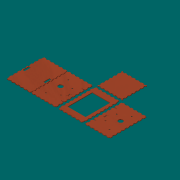
# Autodesk Inventor part: panelsWithKerf
Saved by Autodesk Inventor 2016 SP2 (Build 200236200, 236)
## iProperties
Created: 2016-09-07
Part Number: panelsWithKerf
Material: Generic
Document SubType Name: Modeling
Designer: sawaiz
Density: 1 g/cm^3
Appearance: Copper - Satin
Author: sawaiz
Autodesk Inventor part; units mm, degrees
(part 1 of 2)
ref_plane "YZ Plane" through (0, 0, 0) normal (1, 0, 0) x (0, 1, 0)
ref_plane "XZ Plane" through (0, 0, 0) normal (0, 1, 0) x (-1, 0, 0)
ref_plane "XY Plane" through (0, 0, 0) normal (0, 0, 1) x (1, 0, 0)
sketch "Sketch2" plane through (0, 0, 0) normal (0, 0, 1) x (1, 0, 0)
  line L0 (-285.4, 15) -> (-285.4, -15) construction
  line L1 (-285.4, -15) -> (-295.4, -15) construction
  line L2 (-295.4, -15) -> (-295.4, 15) construction
  line L3 (-295.4, 15) -> (-285.4, 15) construction
  line L4 (-185.4, 15) -> (-185.4, -15) construction
  line L5 (-185.4, -15) -> (-195.4, -15) construction
  line L6 (-195.4, -15) -> (-195.4, 15) construction
  line L7 (-195.4, 15) -> (-185.4, 15) construction
  circle A0 centre (-297.225, -50) radius 1.7 projected
  circle A1 centre (-297.225, 50) radius 1.7 projected
  circle A2 centre (-183.575, -50) radius 1.7 projected
  circle A3 centre (-183.575, 50) radius 1.7 projected
  line L8 (-297.225, 86.825) -> (-297.225, 75) construction
  line L9 (-297.225, 75) -> (-300.4, 75) construction
  line L10 (-300.4, 75) -> (-300.4, 65) construction
  line L11 (-300.4, 65) -> (-297.225, 65) construction
  line L12 (-297.225, 65) -> (-297.225, 55) construction
  line L13 (-297.225, 55) -> (-300.4, 55) construction
  line L14 (-300.4, 55) -> (-300.4, 45) construction
  line L15 (-300.4, 45) -> (-297.225, 45) construction
  line L16 (-297.225, 45) -> (-297.225, 35) construction
  line L17 (-297.225, 35) -> (-300.4, 35) construction
  line L18 (-300.4, 35) -> (-300.4, 25) construction
  line L19 (-300.4, 25) -> (-297.225, 25) construction
  line L20 (-297.225, 25) -> (-297.225, 15) construction
  line L21 (-297.225, 15) -> (-300.4, 15) construction
  line L22 (-300.4, 15) -> (-300.4, 5) construction
  line L23 (-300.4, 5) -> (-297.225, 5) construction
  line L24 (-297.225, 5) -> (-297.225, -5) construction
  line L25 (-297.225, -5) -> (-300.4, -5) construction
  line L26 (-300.4, -5) -> (-300.4, -15) construction
  line L27 (-300.4, -15) -> (-297.225, -15) construction
  line L28 (-297.225, -15) -> (-297.225, -25) construction
  line L29 (-297.225, -25) -> (-300.4, -25) construction
  line L30 (-300.4, -25) -> (-300.4, -35) construction
  line L31 (-300.4, -35) -> (-297.225, -35) construction
  line L32 (-297.225, -35) -> (-297.225, -45) construction
  line L33 (-297.225, -45) -> (-300.4, -45) construction
  line L34 (-300.4, -45) -> (-300.4, -55) construction
  line L35 (-300.4, -55) -> (-297.225, -55) construction
  line L36 (-297.225, -55) -> (-297.225, -65) construction
  line L37 (-297.225, -65) -> (-300.4, -65) construction
  line L38 (-300.4, -65) -> (-300.4, -75) construction
  line L39 (-300.4, -75) -> (-297.225, -75) construction
  line L40 (-297.225, -75) -> (-297.225, -86.825) construction
  line L41 (-297.225, -86.825) -> (-295.4, -86.825) construction
  line L42 (-295.4, -86.825) -> (-295.4, -90) construction
  line L43 (-295.4, -90) -> (-285.4, -90) construction
  line L44 (-285.4, -90) -> (-285.4, -86.825) construction
  line L45 (-285.4, -86.825) -> (-275.4, -86.825) construction
  line L46 (-275.4, -86.825) -> (-275.4, -90) construction
  line L47 (-275.4, -90) -> (-265.4, -90) construction
  line L48 (-265.4, -90) -> (-265.4, -86.825) construction
  line L49 (-265.4, -86.825) -> (-255.4, -86.825) construction
  line L50 (-255.4, -86.825) -> (-255.4, -90) construction
  line L51 (-255.4, -90) -> (-245.4, -90) construction
  line L52 (-245.4, -90) -> (-245.4, -86.825) construction
  line L53 (-245.4, -86.825) -> (-235.4, -86.825) construction
  line L54 (-235.4, -86.825) -> (-235.4, -90) construction
  line L55 (-235.4, -90) -> (-225.4, -90) construction
  line L56 (-225.4, -90) -> (-225.4, -86.825) construction
  line L57 (-225.4, -86.825) -> (-215.4, -86.825) construction
  line L58 (-215.4, -86.825) -> (-215.4, -90) construction
  line L59 (-215.4, -90) -> (-205.4, -90) construction
  line L60 (-205.4, -90) -> (-205.4, -86.825) construction
  line L61 (-205.4, -86.825) -> (-195.4, -86.825) construction
  line L62 (-195.4, -86.825) -> (-195.4, -90) construction
  line L63 (-195.4, -90) -> (-185.4, -90) construction
  line L64 (-185.4, -90) -> (-185.4, -86.825) construction
  line L65 (-185.4, -86.825) -> (-183.575, -86.825) construction
  line L66 (-183.575, -86.825) -> (-183.575, -75) construction
  line L67 (-183.575, -75) -> (-180.4, -75) construction
  line L68 (-180.4, -75) -> (-180.4, -65) construction
  line L69 (-180.4, -65) -> (-183.575, -65) construction
  line L70 (-183.575, -65) -> (-183.575, -55) construction
  line L71 (-183.575, -55) -> (-180.4, -55) construction
  line L72 (-180.4, -55) -> (-180.4, -45) construction
  line L73 (-180.4, -45) -> (-183.575, -45) construction
  line L74 (-183.575, -45) -> (-183.575, -35) construction
  line L75 (-183.575, -35) -> (-180.4, -35) construction
  line L76 (-180.4, -35) -> (-180.4, -25) construction
  line L77 (-180.4, -25) -> (-183.575, -25) construction
  line L78 (-183.575, -25) -> (-183.575, -15) construction
  line L79 (-183.575, -15) -> (-180.4, -15) construction
  line L80 (-180.4, -15) -> (-180.4, -5) construction
  line L81 (-180.4, -5) -> (-183.575, -5) construction
  line L82 (-183.575, -5) -> (-183.575, 5) construction
  line L83 (-183.575, 5) -> (-180.4, 5) construction
  line L84 (-180.4, 5) -> (-180.4, 15) construction
  line L85 (-180.4, 15) -> (-183.575, 15) construction
  line L86 (-183.575, 15) -> (-183.575, 25) construction
  line L87 (-183.575, 25) -> (-180.4, 25) construction
  line L88 (-180.4, 25) -> (-180.4, 35) construction
  line L89 (-180.4, 35) -> (-183.575, 35) construction
  line L90 (-183.575, 35) -> (-183.575, 45) construction
  line L91 (-183.575, 45) -> (-180.4, 45) construction
  line L92 (-180.4, 45) -> (-180.4, 55) construction
  line L93 (-180.4, 55) -> (-183.575, 55) construction
  line L94 (-183.575, 55) -> (-183.575, 65) construction
  line L95 (-183.575, 65) -> (-180.4, 65) construction
  line L96 (-180.4, 65) -> (-180.4, 75) construction
  line L97 (-180.4, 75) -> (-183.575, 75) construction
  line L98 (-183.575, 75) -> (-183.575, 86.825) construction
  line L99 (-183.575, 86.825) -> (-185.4, 86.825) construction
  line L100 (-185.4, 86.825) -> (-185.4, 90) construction
  line L101 (-185.4, 90) -> (-195.4, 90) construction
  line L102 (-195.4, 90) -> (-195.4, 86.825) construction
  line L103 (-195.4, 86.825) -> (-205.4, 86.825) construction
  line L104 (-205.4, 86.825) -> (-205.4, 90) construction
  line L105 (-205.4, 90) -> (-215.4, 90) construction
  line L106 (-215.4, 90) -> (-215.4, 86.825) construction
  line L107 (-215.4, 86.825) -> (-225.4, 86.825) construction
  line L108 (-225.4, 86.825) -> (-225.4, 90) construction
  line L109 (-225.4, 90) -> (-235.4, 90) construction
  line L110 (-235.4, 90) -> (-235.4, 86.825) construction
  line L111 (-235.4, 86.825) -> (-245.4, 86.825) construction
  line L112 (-245.4, 86.825) -> (-245.4, 90) construction
  line L113 (-245.4, 90) -> (-255.4, 90) construction
  line L114 (-255.4, 90) -> (-255.4, 86.825) construction
  line L115 (-255.4, 86.825) -> (-265.4, 86.825) construction
  line L116 (-265.4, 86.825) -> (-265.4, 90) construction
  line L117 (-265.4, 90) -> (-275.4, 90) construction
  line L118 (-275.4, 90) -> (-275.4, 86.825) construction
  line L119 (-275.4, 86.825) -> (-285.4, 86.825) construction
  line L120 (-285.4, 86.825) -> (-285.4, 90) construction
  line L121 (-285.4, 90) -> (-295.4, 90) construction
  line L122 (-295.4, 90) -> (-295.4, 86.825) construction
  line L123 (-295.4, 86.825) -> (-297.225, 86.825) construction
  line L124 (-76.385, -13.335) -> (-80.195, -13.335) projected
  line L125 (-80.195, -13.335) -> (-80.195, -1.905) projected
  line L126 (-80.195, -1.905) -> (-76.385, -1.905) projected
  line L127 (-76.385, -1.905) -> (-76.385, -13.335) projected
  circle A4 centre (-82.1, -15.24) radius 1.078 projected
  circle A5 centre (-74.48, 0) radius 1.078 projected
  circle A6 centre (-74.48, -15.24) radius 1.078 projected
  circle A7 centre (-82.1, 0) radius 1.078 projected
  line L128 (-65.375, -48.5) -> (-63.375, -48.5) construction
  line L129 (-63.375, -48.5) -> (-63.375, -45) construction
  line L130 (-63.375, -45) -> (-60.2, -45) construction
  line L131 (-60.2, -45) -> (-60.2, -35) construction
  line L132 (-60.2, -35) -> (-63.375, -35) construction
  line L133 (-63.375, -35) -> (-63.375, -25) construction
  line L134 (-63.375, -25) -> (-60.2, -25) construction
  line L135 (-60.2, -25) -> (-60.2, -15) construction
  line L136 (-60.2, -15) -> (-63.375, -15) construction
  line L137 (-63.375, -15) -> (-63.375, -5) construction
  line L138 (-63.375, -5) -> (-60.2, -5) construction
  line L139 (-60.2, -5) -> (-60.2, 5) construction
  line L140 (-60.2, 5) -> (-63.375, 5) construction
  line L141 (-63.375, 5) -> (-63.375, 15) construction
  line L142 (-63.375, 15) -> (-60.2, 15) construction
  line L143 (-60.2, 15) -> (-60.2, 25) construction
  line L144 (-60.2, 25) -> (-63.375, 25) construction
  line L145 (-63.375, 25) -> (-63.375, 35) construction
  line L146 (-63.375, 35) -> (-60.2, 35) construction
  line L147 (-60.2, 35) -> (-60.2, 45) construction
  line L148 (-60.2, 45) -> (-63.375, 45) construction
  line L149 (-63.375, 45) -> (-63.375, 48.5) construction
  line L150 (-63.375, 48.5) -> (-65.375, 48.5) construction
  line L151 (-65.375, 48.5) -> (-65.375, 47.25) construction
  line L152 (-65.375, 47.25) -> (-67.875, 47.25) construction
  line L153 (-67.875, 47.25) -> (-67.875, 48.5) construction
  line L154 (-67.875, 48.5) -> (-74.2, 48.5) construction
  line L155 (-74.2, 48.5) -> (-74.2, 51.5) construction
  line L156 (-74.2, 51.5) -> (-67.875, 51.5) construction
  line L157 (-67.875, 51.5) -> (-67.875, 52.75) construction
  line L158 (-67.875, 52.75) -> (-65.375, 52.75) construction
  line L159 (-65.375, 52.75) -> (-65.375, 51.5) construction
  line L160 (-65.375, 51.5) -> (-63.375, 51.5) construction
  line L161 (-63.375, 51.5) -> (-63.375, 55) construction
  line L162 (-63.375, 55) -> (-60.2, 55) construction
  line L163 (-60.2, 55) -> (-60.2, 65) construction
  line L164 (-60.2, 65) -> (-63.375, 65) construction
  line L165 (-63.375, 65) -> (-63.375, 75) construction
  line L166 (-63.375, 75) -> (-60.2, 75) construction
  line L167 (-60.2, 75) -> (-60.2, 86.825) construction
  line L168 (-65.2, 86.825) -> (-60.2, 86.825) construction
  line L169 (-65.2, 90) -> (-65.2, 86.825) construction
  line L170 (-75.2, 90) -> (-65.2, 90) construction
  line L171 (-75.2, 86.825) -> (-75.2, 90) construction
  line L172 (-75.2, 86.825) -> (-85.2, 86.825) construction
  line L173 (-85.2, 90) -> (-85.2, 86.825) construction
  line L174 (-95.2, 90) -> (-85.2, 90) construction
  line L175 (-95.2, 86.825) -> (-95.2, 90) construction
  line L176 (-95.2, 86.825) -> (-105.2, 86.825) construction
  line L177 (-105.2, 90) -> (-105.2, 86.825) construction
  line L178 (-115.2, 90) -> (-105.2, 90) construction
  line L179 (-115.2, 86.825) -> (-115.2, 90) construction
  line L180 (-115.2, 86.825) -> (-125.2, 86.825) construction
  line L181 (-125.2, 90) -> (-125.2, 86.825) construction
  line L182 (-135.2, 90) -> (-125.2, 90) construction
  line L183 (-135.2, 86.825) -> (-135.2, 90) construction
  line L184 (-135.2, 86.825) -> (-145.2, 86.825) construction
  line L185 (-145.2, 90) -> (-145.2, 86.825) construction
  line L186 (-155.2, 90) -> (-145.2, 90) construction
  line L187 (-155.2, 86.825) -> (-155.2, 90) construction
  line L188 (-155.2, 86.825) -> (-165.2, 86.825) construction
  line L189 (-165.2, 90) -> (-165.2, 86.825) construction
  line L190 (-175.2, 90) -> (-165.2, 90) construction
  line L191 (-175.2, 86.825) -> (-175.2, 90) construction
  line L192 (-175.2, 86.825) -> (-180.2, 86.825) construction
  line L193 (-180.2, 75) -> (-180.2, 86.825) construction
  line L194 (-177.025, 75) -> (-180.2, 75) construction
  line L195 (-177.025, 75) -> (-177.025, 65) construction
  line L196 (-180.2, 65) -> (-177.025, 65) construction
  line L197 (-180.2, 55) -> (-180.2, 65) construction
  line L198 (-177.025, 55) -> (-180.2, 55) construction
  line L199 (-177.025, 55) -> (-177.025, 45) construction
  line L200 (-180.2, 45) -> (-177.025, 45) construction
  line L201 (-180.2, 35) -> (-180.2, 45) construction
  line L202 (-177.025, 35) -> (-180.2, 35) construction
  line L203 (-177.025, 35) -> (-177.025, 25) construction
  line L204 (-180.2, 25) -> (-177.025, 25) construction
  line L205 (-180.2, 15) -> (-180.2, 25) construction
  line L206 (-177.025, 15) -> (-180.2, 15) construction
  line L207 (-177.025, 15) -> (-177.025, 5) construction
  line L208 (-180.2, 5) -> (-177.025, 5) construction
  line L209 (-180.2, -5) -> (-180.2, 5) construction
  line L210 (-177.025, -5) -> (-180.2, -5) construction
  line L211 (-177.025, -5) -> (-177.025, -15) construction
  line L212 (-180.2, -15) -> (-177.025, -15) construction
  line L213 (-180.2, -25) -> (-180.2, -15) construction
  line L214 (-177.025, -25) -> (-180.2, -25) construction
  line L215 (-177.025, -25) -> (-177.025, -35) construction
  line L216 (-180.2, -35) -> (-177.025, -35) construction
  line L217 (-180.2, -45) -> (-180.2, -35) construction
  line L218 (-177.025, -45) -> (-180.2, -45) construction
  line L219 (-177.025, -45) -> (-177.025, -55) construction
  line L220 (-180.2, -55) -> (-177.025, -55) construction
  line L221 (-180.2, -65) -> (-180.2, -55) construction
  line L222 (-177.025, -65) -> (-180.2, -65) construction
  line L223 (-177.025, -65) -> (-177.025, -75) construction
  line L224 (-180.2, -75) -> (-177.025, -75) construction
  line L225 (-180.2, -75) -> (-180.2, -86.825) construction
  line L226 (-180.2, -86.825) -> (-175.2, -86.825) construction
  line L227 (-175.2, -86.825) -> (-175.2, -90) construction
  line L228 (-175.2, -90) -> (-165.2, -90) construction
  line L229 (-165.2, -90) -> (-165.2, -86.825) construction
  line L230 (-165.2, -86.825) -> (-155.2, -86.825) construction
  line L231 (-155.2, -86.825) -> (-155.2, -90) construction
  line L232 (-155.2, -90) -> (-145.2, -90) construction
  line L233 (-145.2, -90) -> (-145.2, -86.825) construction
  line L234 (-145.2, -86.825) -> (-135.2, -86.825) construction
  line L235 (-135.2, -86.825) -> (-135.2, -90) construction
  line L236 (-135.2, -90) -> (-125.2, -90) construction
  line L237 (-125.2, -90) -> (-125.2, -86.825) construction
  line L238 (-125.2, -86.825) -> (-115.2, -86.825) construction
  line L239 (-115.2, -86.825) -> (-115.2, -90) construction
  line L240 (-115.2, -90) -> (-105.2, -90) construction
  line L241 (-105.2, -90) -> (-105.2, -86.825) construction
  line L242 (-105.2, -86.825) -> (-95.2, -86.825) construction
  line L243 (-95.2, -86.825) -> (-95.2, -90) construction
  line L244 (-95.2, -90) -> (-85.2, -90) construction
  line L245 (-85.2, -90) -> (-85.2, -86.825) construction
  line L246 (-85.2, -86.825) -> (-75.2, -86.825) construction
  line L247 (-75.2, -86.825) -> (-75.2, -90) construction
  line L248 (-75.2, -90) -> (-65.2, -90) construction
  line L249 (-65.2, -90) -> (-65.2, -86.825) construction
  line L250 (-65.2, -86.825) -> (-60.2, -86.825) construction
  line L251 (-60.2, -86.825) -> (-60.2, -75) construction
  line L252 (-60.2, -75) -> (-63.375, -75) construction
  line L253 (-63.375, -75) -> (-63.375, -65) construction
  line L254 (-63.375, -65) -> (-60.2, -65) construction
  line L255 (-60.2, -65) -> (-60.2, -55) construction
  line L256 (-60.2, -55) -> (-63.375, -55) construction
  line L257 (-63.375, -55) -> (-63.375, -51.5) construction
  line L258 (-63.375, -51.5) -> (-65.375, -51.5) construction
  line L259 (-65.375, -51.5) -> (-65.375, -52.75) construction
  line L260 (-65.375, -52.75) -> (-67.875, -52.75) construction
  line L261 (-67.875, -52.75) -> (-67.875, -51.5) construction
  line L262 (-67.875, -51.5) -> (-74.2, -51.5) construction
  line L263 (-74.2, -51.5) -> (-74.2, -48.5) construction
  line L264 (-74.2, -48.5) -> (-67.875, -48.5) construction
  line L265 (-67.875, -48.5) -> (-67.875, -47.25) construction
  line L266 (-67.875, -47.25) -> (-65.375, -47.25) construction
  line L267 (-65.375, -47.25) -> (-65.375, -48.5) construction
  circle A8 centre (-97.2028, -27.4451) radius 3 projected
  circle A9 centre (-143.1972, 54) radius 3 projected
  circle A10 centre (-97.2028, 27.4451) radius 3 projected
  circle A11 centre (-143.1972, -54) radius 3 projected
  circle A12 centre (-135.2, 8.175) radius 11 projected
  line L268 (43.8, 60) -> (43.8, -60) construction
  line L269 (43.8, -60) -> (-43.8, -60) construction
  line L270 (-43.8, -60) -> (-43.8, 60) construction
  line L271 (-43.8, 60) -> (43.8, 60) construction
  line L272 (-56.825, 86.825) -> (-56.825, 75) construction
  line L273 (-56.825, 75) -> (-60, 75) construction
  line L274 (-60, 75) -> (-60, 65) construction
  line L275 (-60, 65) -> (-56.825, 65) construction
  line L276 (-56.825, 65) -> (-56.825, 55) construction
  line L277 (-56.825, 55) -> (-60, 55) construction
  line L278 (-60, 55) -> (-60, 45) construction
  line L279 (-60, 45) -> (-56.825, 45) construction
  line L280 (-56.825, 45) -> (-56.825, 35) construction
  line L281 (-56.825, 35) -> (-60, 35) construction
  line L282 (-60, 35) -> (-60, 25) construction
  line L283 (-60, 25) -> (-56.825, 25) construction
  line L284 (-56.825, 25) -> (-56.825, 15) construction
  line L285 (-56.825, 15) -> (-60, 15) construction
  line L286 (-60, 15) -> (-60, 5) construction
  line L287 (-60, 5) -> (-56.825, 5) construction
  line L288 (-56.825, 5) -> (-56.825, -5) construction
  line L289 (-56.825, -5) -> (-60, -5) construction
  line L290 (-60, -5) -> (-60, -15) construction
  line L291 (-60, -15) -> (-56.825, -15) construction
  line L292 (-56.825, -15) -> (-56.825, -25) construction
  line L293 (-56.825, -25) -> (-60, -25) construction
  line L294 (-60, -25) -> (-60, -35) construction
  line L295 (-60, -35) -> (-56.825, -35) construction
  line L296 (-56.825, -35) -> (-56.825, -45) construction
  line L297 (-56.825, -45) -> (-60, -45) construction
  line L298 (-60, -45) -> (-60, -55) construction
  line L299 (-60, -55) -> (-56.825, -55) construction
  line L300 (-56.825, -55) -> (-56.825, -65) construction
  line L301 (-56.825, -65) -> (-60, -65) construction
  line L302 (-60, -65) -> (-60, -75) construction
  line L303 (-60, -75) -> (-56.825, -75) construction
  line L304 (-56.825, -75) -> (-56.825, -86.825) construction
  line L305 (-56.825, -86.825) -> (-55, -86.825) construction
  line L306 (-55, -86.825) -> (-55, -90) construction
  line L307 (-55, -90) -> (-45, -90) construction
  line L308 (-45, -90) -> (-45, -86.825) construction
  line L309 (-45, -86.825) -> (-35, -86.825) construction
  line L310 (-35, -86.825) -> (-35, -90) construction
  line L311 (-35, -90) -> (-25, -90) construction
  line L312 (-25, -90) -> (-25, -86.825) construction
  line L313 (-25, -86.825) -> (-15, -86.825) construction
  line L314 (-15, -86.825) -> (-15, -90) construction
  line L315 (-15, -90) -> (-5, -90) construction
  line L316 (-5, -90) -> (-5, -86.825) construction
  line L317 (-5, -86.825) -> (5, -86.825) construction
  line L318 (5, -86.825) -> (5, -90) construction
  line L319 (5, -90) -> (15, -90) construction
  line L320 (15, -90) -> (15, -86.825) construction
  line L321 (15, -86.825) -> (25, -86.825) construction
  line L322 (25, -86.825) -> (25, -90) construction
  line L323 (25, -90) -> (35, -90) construction
  line L324 (35, -90) -> (35, -86.825) construction
  line L325 (35, -86.825) -> (45, -86.825) construction
  line L326 (45, -86.825) -> (45, -90) construction
  line L327 (45, -90) -> (55, -90) construction
  line L328 (55, -90) -> (55, -86.825) construction
  line L329 (55, -86.825) -> (56.825, -86.825) construction
  line L330 (56.825, -86.825) -> (56.825, -75) construction
  line L331 (56.825, -75) -> (60, -75) construction
  line L332 (60, -75) -> (60, -65) construction
  line L333 (60, -65) -> (56.825, -65) construction
  line L334 (56.825, -65) -> (56.825, -55) construction
  line L335 (56.825, -55) -> (60, -55) construction
  line L336 (60, -55) -> (60, -45) construction
  line L337 (60, -45) -> (56.825, -45) construction
  line L338 (56.825, -45) -> (56.825, -35) construction
  line L339 (56.825, -35) -> (60, -35) construction
  line L340 (60, -35) -> (60, -25) construction
  line L341 (60, -25) -> (56.825, -25) construction
  line L342 (56.825, -25) -> (56.825, -15) construction
  line L343 (56.825, -15) -> (60, -15) construction
  line L344 (60, -15) -> (60, -5) construction
  line L345 (60, -5) -> (56.825, -5) construction
  line L346 (56.825, -5) -> (56.825, 5) construction
  line L347 (56.825, 5) -> (60, 5) construction
  line L348 (60, 5) -> (60, 15) construction
  line L349 (60, 15) -> (56.825, 15) construction
  line L350 (56.825, 15) -> (56.825, 25) construction
  line L351 (56.825, 25) -> (60, 25) construction
  line L352 (60, 25) -> (60, 35) construction
  line L353 (60, 35) -> (56.825, 35) construction
  line L354 (56.825, 35) -> (56.825, 45) construction
  line L355 (56.825, 45) -> (60, 45) construction
  line L356 (60, 45) -> (60, 55) construction
  line L357 (60, 55) -> (56.825, 55) construction
  line L358 (56.825, 55) -> (56.825, 65) construction
  line L359 (56.825, 65) -> (60, 65) construction
  line L360 (60, 65) -> (60, 75) construction
  line L361 (60, 75) -> (56.825, 75) construction
  line L362 (56.825, 75) -> (56.825, 86.825) construction
  line L363 (56.825, 86.825) -> (55, 86.825) construction
  line L364 (55, 86.825) -> (55, 90) construction
  line L365 (55, 90) -> (45, 90) construction
  line L366 (45, 90) -> (45, 86.825) construction
  line L367 (45, 86.825) -> (35, 86.825) construction
  line L368 (35, 86.825) -> (35, 90) construction
  line L369 (35, 90) -> (25, 90) construction
  line L370 (25, 90) -> (25, 86.825) construction
  line L371 (25, 86.825) -> (15, 86.825) construction
  line L372 (15, 86.825) -> (15, 90) construction
  line L373 (15, 90) -> (5, 90) construction
  line L374 (5, 90) -> (5, 86.825) construction
  line L375 (5, 86.825) -> (-5, 86.825) construction
  line L376 (-5, 86.825) -> (-5, 90) construction
  line L377 (-5, 90) -> (-15, 90) construction
  line L378 (-15, 90) -> (-15, 86.825) construction
  line L379 (-15, 86.825) -> (-25, 86.825) construction
  line L380 (-25, 86.825) -> (-25, 90) construction
  line L381 (-25, 90) -> (-35, 90) construction
  line L382 (-35, 90) -> (-35, 86.825) construction
  line L383 (-35, 86.825) -> (-45, 86.825) construction
  line L384 (-45, 86.825) -> (-45, 90) construction
  line L385 (-45, 90) -> (-55, 90) construction
  line L386 (-55, 90) -> (-55, 86.825) construction
  line L387 (-55, 86.825) -> (-56.825, 86.825) construction
  line L388 (56.825, 205.2) -> (60, 205.2) construction
  line L389 (60, 205.2) -> (60, 210.2) construction
  line L390 (60, 210.2) -> (55, 210.2) construction
  line L391 (55, 210.2) -> (55, 207.025) construction
  line L392 (55, 207.025) -> (45, 207.025) construction
  line L393 (45, 207.025) -> (45, 210.2) construction
  line L394 (45, 210.2) -> (35, 210.2) construction
  line L395 (35, 210.2) -> (35, 207.025) construction
  line L396 (35, 207.025) -> (25, 207.025) construction
  line L397 (25, 207.025) -> (25, 210.2) construction
  line L398 (25, 210.2) -> (15, 210.2) construction
  line L399 (15, 210.2) -> (15, 207.025) construction
  line L400 (15, 207.025) -> (5, 207.025) construction
  line L401 (5, 207.025) -> (5, 210.2) construction
  line L402 (5, 210.2) -> (-5, 210.2) construction
  line L403 (-5, 210.2) -> (-5, 207.025) construction
  line L404 (-5, 207.025) -> (-15, 207.025) construction
  line L405 (-15, 207.025) -> (-15, 210.2) construction
  line L406 (-15, 210.2) -> (-25, 210.2) construction
  line L407 (-25, 210.2) -> (-25, 207.025) construction
  line L408 (-25, 207.025) -> (-35, 207.025) construction
  line L409 (-35, 207.025) -> (-35, 210.2) construction
  line L410 (-35, 210.2) -> (-45, 210.2) construction
  line L411 (-45, 210.2) -> (-45, 207.025) construction
  line L412 (-45, 207.025) -> (-55, 207.025) construction
  line L413 (-55, 207.025) -> (-55, 210.2) construction
  line L414 (-55, 210.2) -> (-60, 210.2) construction
  line L415 (-60, 210.2) -> (-60, 205.2) construction
  line L416 (-60, 205.2) -> (-56.825, 205.2) construction
  line L417 (-56.825, 205.2) -> (-56.825, 195.2) construction
  line L418 (-56.825, 195.2) -> (-60, 195.2) construction
  line L419 (-60, 195.2) -> (-60, 185.2) construction
  line L420 (-60, 185.2) -> (-56.825, 185.2) construction
  line L421 (-56.825, 185.2) -> (-56.825, 175.2) construction
  line L422 (-56.825, 175.2) -> (-60, 175.2) construction
  line L423 (-60, 175.2) -> (-60, 165.2) construction
  line L424 (-60, 165.2) -> (-56.825, 165.2) construction
  line L425 (-56.825, 165.2) -> (-56.825, 155.2) construction
  line L426 (-56.825, 155.2) -> (-60, 155.2) construction
  line L427 (-60, 155.2) -> (-60, 145.2) construction
  line L428 (-60, 145.2) -> (-56.825, 145.2) construction
  line L429 (-56.825, 145.2) -> (-56.825, 135.2) construction
  line L430 (-56.825, 135.2) -> (-60, 135.2) construction
  line L431 (-60, 135.2) -> (-60, 125.2) construction
  line L432 (-60, 125.2) -> (-56.825, 125.2) construction
  line L433 (-56.825, 125.2) -> (-56.825, 115.2) construction
  line L434 (-56.825, 115.2) -> (-60, 115.2) construction
  line L435 (-60, 115.2) -> (-60, 105.2) construction
  line L436 (-60, 105.2) -> (-56.825, 105.2) construction
  line L437 (-56.825, 105.2) -> (-56.825, 95.2) construction
  line L438 (-56.825, 95.2) -> (-60, 95.2) construction
  line L439 (-60, 95.2) -> (-60, 90.2) construction
  line L440 (-60, 90.2) -> (-55, 90.2) construction
  line L441 (-55, 90.2) -> (-55, 93.375) construction
  line L442 (-55, 93.375) -> (-45, 93.375) construction
  line L443 (-45, 93.375) -> (-45, 90.2) construction
  line L444 (-45, 90.2) -> (-35, 90.2) construction
  line L445 (-35, 90.2) -> (-35, 93.375) construction
  line L446 (-35, 93.375) -> (-25, 93.375) construction
  line L447 (-25, 93.375) -> (-25, 90.2) construction
  line L448 (-25, 90.2) -> (-15, 90.2) construction
  line L449 (-15, 90.2) -> (-15, 93.375) construction
  line L450 (-15, 93.375) -> (-5, 93.375) construction
  line L451 (-5, 93.375) -> (-5, 90.2) construction
  line L452 (-5, 90.2) -> (5, 90.2) construction
  line L453 (5, 90.2) -> (5, 93.375) construction
  line L454 (5, 93.375) -> (15, 93.375) construction
  line L455 (15, 93.375) -> (15, 90.2) construction
  line L456 (15, 90.2) -> (25, 90.2) construction
  line L457 (25, 90.2) -> (25, 93.375) construction
  line L458 (25, 93.375) -> (35, 93.375) construction
  line L459 (35, 93.375) -> (35, 90.2) construction
  line L460 (35, 90.2) -> (45, 90.2) construction
  line L461 (45, 90.2) -> (45, 93.375) construction
  line L462 (45, 93.375) -> (55, 93.375) construction
  line L463 (55, 93.375) -> (55, 90.2) construction
  line L464 (55, 90.2) -> (60, 90.2) construction
  line L465 (60, 90.2) -> (60, 95.2) construction
  line L466 (60, 95.2) -> (56.825, 95.2) construction
  line L467 (56.825, 95.2) -> (56.825, 105.2) construction
  line L468 (56.825, 105.2) -> (60, 105.2) construction
  line L469 (60, 105.2) -> (60, 115.2) construction
  line L470 (60, 115.2) -> (56.825, 115.2) construction
  line L471 (56.825, 115.2) -> (56.825, 125.2) construction
  line L472 (56.825, 125.2) -> (60, 125.2) construction
  line L473 (60, 125.2) -> (60, 135.2) construction
  line L474 (60, 135.2) -> (56.825, 135.2) construction
  line L475 (56.825, 135.2) -> (56.825, 145.2) construction
  line L476 (56.825, 145.2) -> (60, 145.2) construction
  line L477 (60, 145.2) -> (60, 155.2) construction
  line L478 (60, 155.2) -> (56.825, 155.2) construction
  line L479 (56.825, 155.2) -> (56.825, 165.2) construction
  line L480 (56.825, 165.2) -> (60, 165.2) construction
  line L481 (60, 165.2) -> (60, 175.2) construction
  line L482 (60, 175.2) -> (56.825, 175.2) construction
  line L483 (56.825, 175.2) -> (56.825, 185.2) construction
  line L484 (56.825, 185.2) -> (60, 185.2) construction
  line L485 (60, 185.2) -> (60, 195.2) construction
  line L486 (60, 195.2) -> (56.825, 195.2) construction
  line L487 (56.825, 195.2) -> (56.825, 205.2) construction
  line L488 (80.195, -13.335) -> (76.385, -13.335) projected
  line L489 (76.385, -13.335) -> (76.385, -1.905) projected
  line L490 (76.385, -1.905) -> (80.195, -1.905) projected
  line L491 (80.195, -1.905) -> (80.195, -13.335) projected
  circle A13 centre (82.1, -15.24) radius 1.078 projected
  circle A14 centre (74.48, 0) radius 1.078 projected
  circle A15 centre (74.48, -15.24) radius 1.078 projected
  circle A16 centre (82.1, 0) radius 1.078 projected
  circle A17 centre (97.2028, -27.4451) radius 3 projected
  circle A18 centre (143.1972, 54) radius 3 projected
  circle A19 centre (97.2028, 27.4451) radius 3 projected
  circle A20 centre (143.1972, -54) radius 3 projected
  circle A21 centre (135.2, 8.175) radius 11 projected
  line L492 (63.375, -48.5) -> (65.375, -48.5) construction
  line L493 (65.375, -48.5) -> (65.375, -47.25) construction
  line L494 (65.375, -47.25) -> (67.875, -47.25) construction
  line L495 (67.875, -47.25) -> (67.875, -48.5) construction
  line L496 (67.875, -48.5) -> (74.2, -48.5) construction
  line L497 (74.2, -48.5) -> (74.2, -51.5) construction
  line L498 (74.2, -51.5) -> (67.875, -51.5) construction
  line L499 (67.875, -51.5) -> (67.875, -52.75) construction
  line L500 (67.875, -52.75) -> (65.375, -52.75) construction
  line L501 (65.375, -52.75) -> (65.375, -51.5) construction
  line L502 (65.375, -51.5) -> (63.375, -51.5) construction
  line L503 (63.375, -55) -> (63.375, -51.5) construction
  line L504 (60.2, -55) -> (63.375, -55) construction
  line L505 (60.2, -65) -> (60.2, -55) construction
  line L506 (63.375, -65) -> (60.2, -65) construction
  line L507 (63.375, -75) -> (63.375, -65) construction
  line L508 (60.2, -75) -> (63.375, -75) construction
  line L509 (60.2, -86.825) -> (60.2, -75) construction
  line L510 (65.2, -86.825) -> (60.2, -86.825) construction
  line L511 (65.2, -90) -> (65.2, -86.825) construction
  line L512 (75.2, -90) -> (65.2, -90) construction
  line L513 (75.2, -86.825) -> (75.2, -90) construction
  line L514 (85.2, -86.825) -> (75.2, -86.825) construction
  line L515 (85.2, -90) -> (85.2, -86.825) construction
  line L516 (95.2, -90) -> (85.2, -90) construction
  line L517 (95.2, -86.825) -> (95.2, -90) construction
  line L518 (105.2, -86.825) -> (95.2, -86.825) construction
  line L519 (105.2, -90) -> (105.2, -86.825) construction
  line L520 (115.2, -90) -> (105.2, -90) construction
  line L521 (115.2, -86.825) -> (115.2, -90) construction
  line L522 (125.2, -86.825) -> (115.2, -86.825) construction
  line L523 (125.2, -90) -> (125.2, -86.825) construction
  line L524 (135.2, -90) -> (125.2, -90) construction
  line L525 (135.2, -86.825) -> (135.2, -90) construction
  line L526 (145.2, -86.825) -> (135.2, -86.825) construction
  line L527 (145.2, -90) -> (145.2, -86.825) construction
  line L528 (155.2, -90) -> (145.2, -90) construction
  line L529 (155.2, -86.825) -> (155.2, -90) construction
  line L530 (165.2, -86.825) -> (155.2, -86.825) construction
  line L531 (165.2, -90) -> (165.2, -86.825) construction
  line L532 (175.2, -90) -> (165.2, -90) construction
  line L533 (175.2, -86.825) -> (175.2, -90) construction
  line L534 (180.2, -86.825) -> (175.2, -86.825) construction
  line L535 (180.2, -86.825) -> (180.2, -75) construction
  line L536 (180.2, -75) -> (177.025, -75) construction
  line L537 (177.025, -65) -> (177.025, -75) construction
  line L538 (177.025, -65) -> (180.2, -65) construction
  line L539 (180.2, -65) -> (180.2, -55) construction
  line L540 (180.2, -55) -> (177.025, -55) construction
  line L541 (177.025, -45) -> (177.025, -55) construction
  line L542 (177.025, -45) -> (180.2, -45) construction
  line L543 (180.2, -45) -> (180.2, -35) construction
  line L544 (180.2, -35) -> (177.025, -35) construction
  line L545 (177.025, -25) -> (177.025, -35) construction
  line L546 (177.025, -25) -> (180.2, -25) construction
  line L547 (180.2, -25) -> (180.2, -15) construction
  line L548 (180.2, -15) -> (177.025, -15) construction
  line L549 (177.025, -5) -> (177.025, -15) construction
  line L550 (177.025, -5) -> (180.2, -5) construction
  line L551 (180.2, -5) -> (180.2, 5) construction
  line L552 (180.2, 5) -> (177.025, 5) construction
  line L553 (177.025, 15) -> (177.025, 5) construction
  line L554 (177.025, 15) -> (180.2, 15) construction
  line L555 (180.2, 15) -> (180.2, 25) construction
  line L556 (180.2, 25) -> (177.025, 25) construction
  line L557 (177.025, 35) -> (177.025, 25) construction
  line L558 (177.025, 35) -> (180.2, 35) construction
  line L559 (180.2, 35) -> (180.2, 45) construction
  line L560 (180.2, 45) -> (177.025, 45) construction
  line L561 (177.025, 55) -> (177.025, 45) construction
  line L562 (177.025, 55) -> (180.2, 55) construction
  line L563 (180.2, 55) -> (180.2, 65) construction
  line L564 (180.2, 65) -> (177.025, 65) construction
  line L565 (177.025, 75) -> (177.025, 65) construction
  line L566 (177.025, 75) -> (180.2, 75) construction
  line L567 (180.2, 75) -> (180.2, 86.825) construction
  line L568 (175.2, 86.825) -> (180.2, 86.825) construction
  line L569 (175.2, 86.825) -> (175.2, 90) construction
  line L570 (175.2, 90) -> (165.2, 90) construction
  line L571 (165.2, 90) -> (165.2, 86.825) construction
  line L572 (155.2, 86.825) -> (165.2, 86.825) construction
  line L573 (155.2, 86.825) -> (155.2, 90) construction
  line L574 (155.2, 90) -> (145.2, 90) construction
  line L575 (145.2, 90) -> (145.2, 86.825) construction
  line L576 (135.2, 86.825) -> (145.2, 86.825) construction
  line L577 (135.2, 86.825) -> (135.2, 90) construction
  line L578 (135.2, 90) -> (125.2, 90) construction
  line L579 (125.2, 90) -> (125.2, 86.825) construction
  line L580 (115.2, 86.825) -> (125.2, 86.825) construction
  line L581 (115.2, 86.825) -> (115.2, 90) construction
  line L582 (115.2, 90) -> (105.2, 90) construction
  line L583 (105.2, 90) -> (105.2, 86.825) construction
  line L584 (95.2, 86.825) -> (105.2, 86.825) construction
  line L585 (95.2, 86.825) -> (95.2, 90) construction
  line L586 (95.2, 90) -> (85.2, 90) construction
  line L587 (85.2, 90) -> (85.2, 86.825) construction
  line L588 (75.2, 86.825) -> (85.2, 86.825) construction
  line L589 (75.2, 86.825) -> (75.2, 90) construction
  line L590 (75.2, 90) -> (65.2, 90) construction
  line L591 (65.2, 90) -> (65.2, 86.825) construction
  line L592 (60.2, 86.825) -> (65.2, 86.825) construction
  line L593 (60.2, 75) -> (60.2, 86.825) construction
  line L594 (63.375, 75) -> (60.2, 75) construction
  line L595 (63.375, 65) -> (63.375, 75) construction
  line L596 (60.2, 65) -> (63.375, 65) construction
  line L597 (60.2, 55) -> (60.2, 65) construction
  line L598 (63.375, 55) -> (60.2, 55) construction
  line L599 (63.375, 51.5) -> (63.375, 55) construction
  line L600 (63.375, 51.5) -> (65.375, 51.5) construction
  line L601 (65.375, 51.5) -> (65.375, 52.75) construction
  line L602 (65.375, 52.75) -> (67.875, 52.75) construction
  line L603 (67.875, 52.75) -> (67.875, 51.5) construction
  line L604 (67.875, 51.5) -> (74.2, 51.5) construction
  line L605 (74.2, 51.5) -> (74.2, 48.5) construction
  line L606 (74.2, 48.5) -> (67.875, 48.5) construction
  line L607 (67.875, 48.5) -> (67.875, 47.25) construction
  line L608 (67.875, 47.25) -> (65.375, 47.25) construction
  line L609 (65.375, 47.25) -> (65.375, 48.5) construction
  line L610 (65.375, 48.5) -> (63.375, 48.5) construction
  line L611 (63.375, 45) -> (63.375, 48.5) construction
  line L612 (60.2, 45) -> (63.375, 45) construction
  line L613 (60.2, 35) -> (60.2, 45) construction
  line L614 (63.375, 35) -> (60.2, 35) construction
  line L615 (63.375, 25) -> (63.375, 35) construction
  line L616 (60.2, 25) -> (63.375, 25) construction
  line L617 (60.2, 15) -> (60.2, 25) construction
  line L618 (63.375, 15) -> (60.2, 15) construction
  line L619 (63.375, 5) -> (63.375, 15) construction
  line L620 (60.2, 5) -> (63.375, 5) construction
  line L621 (60.2, -5) -> (60.2, 5) construction
  line L622 (63.375, -5) -> (60.2, -5) construction
  line L623 (63.375, -15) -> (63.375, -5) construction
  line L624 (60.2, -15) -> (63.375, -15) construction
  line L625 (60.2, -25) -> (60.2, -15) construction
  line L626 (63.375, -25) -> (60.2, -25) construction
  line L627 (63.375, -35) -> (63.375, -25) construction
  line L628 (60.2, -35) -> (63.375, -35) construction
  line L629 (60.2, -45) -> (60.2, -35) construction
  line L630 (63.375, -45) -> (60.2, -45) construction
  line L631 (63.375, -48.5) -> (63.375, -45) construction
  line L632 (-297.325, 75.1) -> (-297.325, 86.925)
  line L633 (-297.325, 86.925) -> (-295.5, 86.925)
  line L634 (-295.5, 86.925) -> (-295.5, 90.1)
  line L635 (-295.5, 90.1) -> (-285.3, 90.1)
  line L636 (-285.3, 90.1) -> (-285.3, 86.925)
  line L637 (-285.3, 86.925) -> (-275.5, 86.925)
  line L638 (-275.5, 86.925) -> (-275.5, 90.1)
  line L639 (-275.5, 90.1) -> (-265.3, 90.1)
  line L640 (-265.3, 90.1) -> (-265.3, 86.925)
  line L641 (-265.3, 86.925) -> (-255.5, 86.925)
  line L642 (-255.5, 86.925) -> (-255.5, 90.1)
  line L643 (-255.5, 90.1) -> (-245.3, 90.1)
  line L644 (-245.3, 90.1) -> (-245.3, 86.925)
  line L645 (-245.3, 86.925) -> (-235.5, 86.925)
  line L646 (-235.5, 86.925) -> (-235.5, 90.1)
  line L647 (-235.5, 90.1) -> (-225.3, 90.1)
  line L648 (-225.3, 90.1) -> (-225.3, 86.925)
  line L649 (-225.3, 86.925) -> (-215.5, 86.925)
  line L650 (-215.5, 86.925) -> (-215.5, 90.1)
  line L651 (-215.5, 90.1) -> (-205.3, 90.1)
  line L652 (-205.3, 90.1) -> (-205.3, 86.925)
  line L653 (-205.3, 86.925) -> (-195.5, 86.925)
  line L654 (-195.5, 86.925) -> (-195.5, 90.1)
  line L655 (-195.5, 90.1) -> (-185.3, 90.1)
  line L656 (-185.3, 90.1) -> (-185.3, 86.925)
  line L657 (-185.3, 86.925) -> (-183.475, 86.925)
  line L658 (-183.475, 86.925) -> (-183.475, 75.1)
  line L659 (-183.475, 75.1) -> (-180.3, 75.1)
  line L660 (-180.3, 75.1) -> (-180.3, 64.9)
  line L661 (-180.3, 64.9) -> (-183.475, 64.9)
  line L662 (-183.475, 64.9) -> (-183.475, 55.1)
  line L663 (-183.475, 55.1) -> (-180.3, 55.1)
  line L664 (-180.3, 55.1) -> (-180.3, 44.9)
  line L665 (-180.3, 44.9) -> (-183.475, 44.9)
  line L666 (-183.475, 44.9) -> (-183.475, 35.1)
  line L667 (-183.475, 35.1) -> (-180.3, 35.1)
  line L668 (-180.3, 35.1) -> (-180.3, 24.9)
  line L669 (-180.3, 24.9) -> (-183.475, 24.9)
  line L670 (-183.475, 24.9) -> (-183.475, 15.1)
  line L671 (-183.475, 15.1) -> (-180.3, 15.1)
  line L672 (-180.3, 15.1) -> (-180.3, 4.9)
  line L673 (-180.3, 4.9) -> (-183.475, 4.9)
  line L674 (-183.475, 4.9) -> (-183.475, -4.9)
  line L675 (-183.475, -4.9) -> (-180.3, -4.9)
  line L676 (-180.3, -4.9) -> (-180.3, -15.1)
  line L677 (-180.3, -15.1) -> (-183.475, -15.1)
  line L678 (-183.475, -15.1) -> (-183.475, -24.9)
  line L679 (-183.475, -24.9) -> (-180.3, -24.9)
  line L680 (-180.3, -24.9) -> (-180.3, -35.1)
  line L681 (-180.3, -35.1) -> (-183.475, -35.1)
  line L682 (-183.475, -35.1) -> (-183.475, -44.9)
  line L683 (-183.475, -44.9) -> (-180.3, -44.9)
  line L684 (-180.3, -44.9) -> (-180.3, -55.1)
  line L685 (-180.3, -55.1) -> (-183.475, -55.1)
  line L686 (-183.475, -55.1) -> (-183.475, -64.9)
  line L687 (-183.475, -64.9) -> (-180.3, -64.9)
  line L688 (-180.3, -64.9) -> (-180.3, -75.1)
  line L689 (-180.3, -75.1) -> (-183.475, -75.1)
  line L690 (-183.475, -75.1) -> (-183.475, -86.925)
  line L691 (-183.475, -86.925) -> (-185.3, -86.925)
  line L692 (-185.3, -86.925) -> (-185.3, -90.1)
  line L693 (-185.3, -90.1) -> (-195.5, -90.1)
  line L694 (-195.5, -90.1) -> (-195.5, -86.925)
  line L695 (-195.5, -86.925) -> (-205.3, -86.925)
  line L696 (-205.3, -86.925) -> (-205.3, -90.1)
  line L697 (-205.3, -90.1) -> (-215.5, -90.1)
  line L698 (-215.5, -90.1) -> (-215.5, -86.925)
  line L699 (-215.5, -86.925) -> (-225.3, -86.925)
  line L700 (-225.3, -86.925) -> (-225.3, -90.1)
  line L701 (-225.3, -90.1) -> (-235.5, -90.1)
  line L702 (-235.5, -90.1) -> (-235.5, -86.925)
  line L703 (-235.5, -86.925) -> (-245.3, -86.925)
  line L704 (-245.3, -86.925) -> (-245.3, -90.1)
  line L705 (-245.3, -90.1) -> (-255.5, -90.1)
  line L706 (-255.5, -90.1) -> (-255.5, -86.925)
  line L707 (-255.5, -86.925) -> (-265.3, -86.925)
  line L708 (-265.3, -86.925) -> (-265.3, -90.1)
  line L709 (-265.3, -90.1) -> (-275.5, -90.1)
  line L710 (-275.5, -90.1) -> (-275.5, -86.925)
  line L711 (-275.5, -86.925) -> (-285.3, -86.925)
  line L712 (-285.3, -86.925) -> (-285.3, -90.1)
  line L713 (-285.3, -90.1) -> (-295.5, -90.1)
  line L714 (-295.5, -90.1) -> (-295.5, -86.925)
  line L715 (-295.5, -86.925) -> (-297.325, -86.925)
  line L716 (-297.325, -86.925) -> (-297.325, -75.1)
  line L717 (-297.325, -75.1) -> (-300.5, -75.1)
  line L718 (-300.5, -75.1) -> (-300.5, -64.9)
  line L719 (-300.5, -64.9) -> (-297.325, -64.9)
  line L720 (-297.325, -64.9) -> (-297.325, -55.1)
  line L721 (-297.325, -55.1) -> (-300.5, -55.1)
  line L722 (-300.5, -55.1) -> (-300.5, -44.9)
  line L723 (-300.5, -44.9) -> (-297.325, -44.9)
  line L724 (-297.325, -44.9) -> (-297.325, -35.1)
  line L725 (-297.325, -35.1) -> (-300.5, -35.1)
  line L726 (-300.5, -35.1) -> (-300.5, -24.9)
  line L727 (-300.5, -24.9) -> (-297.325, -24.9)
  line L728 (-297.325, -24.9) -> (-297.325, -15.1)
  line L729 (-297.325, -15.1) -> (-300.5, -15.1)
  line L730 (-300.5, -15.1) -> (-300.5, -4.9)
  line L731 (-300.5, -4.9) -> (-297.325, -4.9)
  line L732 (-297.325, -4.9) -> (-297.325, 4.9)
  line L733 (-297.325, 4.9) -> (-300.5, 4.9)
  line L734 (-300.5, 4.9) -> (-300.5, 15.1)
  line L735 (-300.5, 15.1) -> (-297.325, 15.1)
  line L736 (-297.325, 15.1) -> (-297.325, 24.9)
  line L737 (-297.325, 24.9) -> (-300.5, 24.9)
  line L738 (-300.5, 24.9) -> (-300.5, 35.1)
  line L739 (-300.5, 35.1) -> (-297.325, 35.1)
  line L740 (-297.325, 35.1) -> (-297.325, 44.9)
  line L741 (-297.325, 44.9) -> (-300.5, 44.9)
  line L742 (-300.5, 44.9) -> (-300.5, 55.1)
  line L743 (-300.5, 55.1) -> (-297.325, 55.1)
  line L744 (-297.325, 55.1) -> (-297.325, 64.9)
  line L745 (-297.325, 64.9) -> (-300.5, 64.9)
  line L746 (-300.5, 64.9) -> (-300.5, 75.1)
  line L747 (-300.5, 75.1) -> (-297.325, 75.1)
  line L748 (-285.5, -14.9) -> (-285.5, 14.9)
  line L749 (-285.5, 14.9) -> (-295.3, 14.9)
  line L750 (-295.3, 14.9) -> (-295.3, -14.9)
  line L751 (-295.3, -14.9) -> (-285.5, -14.9)
  line L752 (-195.3, 14.9) -> (-195.3, -14.9)
  line L753 (-195.3, -14.9) -> (-185.5, -14.9)
  line L754 (-185.5, -14.9) -> (-185.5, 14.9)
  line L755 (-185.5, 14.9) -> (-195.3, 14.9)
  line L756 (-165.1, 86.925) -> (-155.3, 86.925)
  line L757 (-155.3, 86.925) -> (-155.3, 90.1)
  line L758 (-155.3, 90.1) -> (-145.1, 90.1)
  line L759 (-145.1, 90.1) -> (-145.1, 86.925)
  line L760 (-145.1, 86.925) -> (-135.3, 86.925)
  line L761 (-135.3, 86.925) -> (-135.3, 90.1)
  line L762 (-135.3, 90.1) -> (-125.1, 90.1)
  line L763 (-125.1, 90.1) -> (-125.1, 86.925)
  line L764 (-125.1, 86.925) -> (-115.3, 86.925)
  line L765 (-115.3, 86.925) -> (-115.3, 90.1)
  line L766 (-115.3, 90.1) -> (-105.1, 90.1)
  line L767 (-105.1, 90.1) -> (-105.1, 86.925)
  line L768 (-105.1, 86.925) -> (-95.3, 86.925)
  line L769 (-95.3, 86.925) -> (-95.3, 90.1)
  line L770 (-95.3, 90.1) -> (-85.1, 90.1)
  line L771 (-85.1, 90.1) -> (-85.1, 86.925)
  line L772 (-85.1, 86.925) -> (-75.3, 86.925)
  line L773 (-75.3, 86.925) -> (-75.3, 90.1)
  line L774 (-75.3, 90.1) -> (-65.1, 90.1)
  line L775 (-65.1, 90.1) -> (-65.1, 86.925)
  line L776 (-65.1, 86.925) -> (-60.1, 86.925)
  line L777 (-60.1, 86.925) -> (-60.1, 74.9)
  line L778 (-60.1, 74.9) -> (-63.275, 74.9)
  line L779 (-63.275, 74.9) -> (-63.275, 65.1)
  line L780 (-63.275, 65.1) -> (-60.1, 65.1)
  line L781 (-60.1, 65.1) -> (-60.1, 54.9)
  line L782 (-60.1, 54.9) -> (-63.275, 54.9)
  line L783 (-63.275, 54.9) -> (-63.275, 51.4)
  line L784 (-63.275, 51.4) -> (-65.475, 51.4)
  line L785 (-65.475, 51.4) -> (-65.475, 52.65)
  line L786 (-65.475, 52.65) -> (-67.775, 52.65)
  line L787 (-67.775, 52.65) -> (-67.775, 51.4)
  line L788 (-67.775, 51.4) -> (-74.1, 51.4)
  line L789 (-74.1, 51.4) -> (-74.1, 48.6)
  line L790 (-74.1, 48.6) -> (-67.775, 48.6)
  line L791 (-67.775, 48.6) -> (-67.775, 47.35)
  line L792 (-67.775, 47.35) -> (-65.475, 47.35)
  line L793 (-65.475, 47.35) -> (-65.475, 48.6)
  line L794 (-65.475, 48.6) -> (-63.275, 48.6)
  line L795 (-63.275, 48.6) -> (-63.275, 45.1)
  line L796 (-63.275, 45.1) -> (-60.1, 45.1)
  line L797 (-60.1, 45.1) -> (-60.1, 34.9)
  line L798 (-60.1, 34.9) -> (-63.275, 34.9)
  line L799 (-63.275, 34.9) -> (-63.275, 25.1)
  line L800 (-63.275, 25.1) -> (-60.1, 25.1)
  line L801 (-60.1, 25.1) -> (-60.1, 14.9)
  line L802 (-60.1, 14.9) -> (-63.275, 14.9)
  line L803 (-63.275, 14.9) -> (-63.275, 5.1)
  line L804 (-63.275, 5.1) -> (-60.1, 5.1)
  line L805 (-60.1, 5.1) -> (-60.1, -5.1)
  line L806 (-60.1, -5.1) -> (-63.275, -5.1)
  line L807 (-63.275, -5.1) -> (-63.275, -14.9)
  line L808 (-63.275, -14.9) -> (-60.1, -14.9)
  line L809 (-60.1, -14.9) -> (-60.1, -25.1)
  line L810 (-60.1, -25.1) -> (-63.275, -25.1)
  line L811 (-63.275, -25.1) -> (-63.275, -34.9)
  line L812 (-63.275, -34.9) -> (-60.1, -34.9)
  line L813 (-60.1, -34.9) -> (-60.1, -45.1)
  line L814 (-60.1, -45.1) -> (-63.275, -45.1)
  line L815 (-63.275, -45.1) -> (-63.275, -48.6)
  line L816 (-63.275, -48.6) -> (-65.475, -48.6)
  line L817 (-65.475, -48.6) -> (-65.475, -47.35)
  line L818 (-65.475, -47.35) -> (-67.775, -47.35)
  line L819 (-67.775, -47.35) -> (-67.775, -48.6)
  line L820 (-67.775, -48.6) -> (-74.1, -48.6)
  line L821 (-74.1, -48.6) -> (-74.1, -51.4)
  line L822 (-74.1, -51.4) -> (-67.775, -51.4)
  line L823 (-67.775, -51.4) -> (-67.775, -52.65)
  line L824 (-67.775, -52.65) -> (-65.475, -52.65)
  line L825 (-65.475, -52.65) -> (-65.475, -51.4)
  line L826 (-65.475, -51.4) -> (-63.275, -51.4)
  line L827 (-63.275, -51.4) -> (-63.275, -54.9)
  line L828 (-63.275, -54.9) -> (-60.1, -54.9)
  line L829 (-60.1, -54.9) -> (-60.1, -65.1)
  line L830 (-60.1, -65.1) -> (-63.275, -65.1)
  line L831 (-63.275, -65.1) -> (-63.275, -74.9)
  line L832 (-63.275, -74.9) -> (-60.1, -74.9)
  line L833 (-60.1, -74.9) -> (-60.1, -86.925)
  line L834 (-60.1, -86.925) -> (-65.1, -86.925)
  line L835 (-65.1, -86.925) -> (-65.1, -90.1)
  line L836 (-65.1, -90.1) -> (-75.3, -90.1)
  line L837 (-75.3, -90.1) -> (-75.3, -86.925)
  line L838 (-75.3, -86.925) -> (-85.1, -86.925)
  line L839 (-85.1, -86.925) -> (-85.1, -90.1)
  line L840 (-85.1, -90.1) -> (-95.3, -90.1)
  line L841 (-95.3, -90.1) -> (-95.3, -86.925)
  line L842 (-95.3, -86.925) -> (-105.1, -86.925)
  line L843 (-105.1, -86.925) -> (-105.1, -90.1)
  line L844 (-105.1, -90.1) -> (-115.3, -90.1)
  line L845 (-115.3, -90.1) -> (-115.3, -86.925)
  line L846 (-115.3, -86.925) -> (-125.1, -86.925)
  line L847 (-125.1, -86.925) -> (-125.1, -90.1)
  line L848 (-125.1, -90.1) -> (-135.3, -90.1)
  line L849 (-135.3, -90.1) -> (-135.3, -86.925)
  line L850 (-135.3, -86.925) -> (-145.1, -86.925)
  line L851 (-145.1, -86.925) -> (-145.1, -90.1)
  line L852 (-145.1, -90.1) -> (-155.3, -90.1)
  line L853 (-155.3, -90.1) -> (-155.3, -86.925)
  line L854 (-155.3, -86.925) -> (-165.1, -86.925)
  line L855 (-165.1, -86.925) -> (-165.1, -90.1)
  line L856 (-165.1, -90.1) -> (-175.3, -90.1)
  line L857 (-175.3, -90.1) -> (-175.3, -86.925)
  line L858 (-175.3, -86.925) -> (-180.3, -86.925)
  line L859 (-180.3, -86.925) -> (-180.3, -74.9)
  line L860 (-180.3, -74.9) -> (-177.125, -74.9)
  line L861 (-177.125, -74.9) -> (-177.125, -65.1)
  line L862 (-177.125, -65.1) -> (-180.3, -65.1)
  line L863 (-180.3, -65.1) -> (-180.3, -54.9)
  line L864 (-180.3, -54.9) -> (-177.125, -54.9)
  line L865 (-177.125, -54.9) -> (-177.125, -45.1)
  line L866 (-177.125, -45.1) -> (-180.3, -45.1)
  line L867 (-180.3, -45.1) -> (-180.3, -34.9)
  line L868 (-180.3, -34.9) -> (-177.125, -34.9)
  line L869 (-177.125, -34.9) -> (-177.125, -25.1)
  line L870 (-177.125, -25.1) -> (-180.3, -25.1)
  line L871 (-180.3, -25.1) -> (-180.3, -14.9)
  line L872 (-180.3, -14.9) -> (-177.125, -14.9)
  line L873 (-177.125, -14.9) -> (-177.125, -5.1)
  line L874 (-177.125, -5.1) -> (-180.3, -5.1)
  line L875 (-180.3, -5.1) -> (-180.3, 5.1)
  line L876 (-180.3, 5.1) -> (-177.125, 5.1)
  line L877 (-177.125, 5.1) -> (-177.125, 14.9)
  line L878 (-177.125, 14.9) -> (-180.3, 14.9)
  line L879 (-180.3, 14.9) -> (-180.3, 25.1)
  line L880 (-180.3, 25.1) -> (-177.125, 25.1)
  line L881 (-177.125, 25.1) -> (-177.125, 34.9)
  line L882 (-177.125, 34.9) -> (-180.3, 34.9)
  line L883 (-180.3, 34.9) -> (-180.3, 45.1)
  line L884 (-180.3, 45.1) -> (-177.125, 45.1)
  line L885 (-177.125, 45.1) -> (-177.125, 54.9)
  line L886 (-177.125, 54.9) -> (-180.3, 54.9)
  line L887 (-180.3, 54.9) -> (-180.3, 65.1)
  line L888 (-180.3, 65.1) -> (-177.125, 65.1)
  line L889 (-177.125, 65.1) -> (-177.125, 74.9)
  line L890 (-177.125, 74.9) -> (-180.3, 74.9)
  line L891 (-180.3, 74.9) -> (-180.3, 86.925)
  line L892 (-180.3, 86.925) -> (-175.3, 86.925)
  line L893 (-175.3, 86.925) -> (-175.3, 90.1)
  line L894 (-175.3, 90.1) -> (-165.1, 90.1)
  line L895 (-165.1, 90.1) -> (-165.1, 86.925)
  line L896 (-15.1, 90.1) -> (-4.9, 90.1)
  line L897 (-4.9, 90.1) -> (-4.9, 86.925)
  line L898 (-4.9, 86.925) -> (4.9, 86.925)
  line L899 (4.9, 86.925) -> (4.9, 90.1)
  line L900 (4.9, 90.1) -> (15.1, 90.1)
  line L901 (15.1, 90.1) -> (15.1, 86.925)
  line L902 (15.1, 86.925) -> (24.9, 86.925)
  line L903 (24.9, 86.925) -> (24.9, 90.1)
  line L904 (24.9, 90.1) -> (35.1, 90.1)
  line L905 (35.1, 90.1) -> (35.1, 86.925)
  line L906 (35.1, 86.925) -> (44.9, 86.925)
  line L907 (44.9, 86.925) -> (44.9, 90.1)
  line L908 (44.9, 90.1) -> (55.1, 90.1)
  line L909 (55.1, 90.1) -> (55.1, 86.925)
  line L910 (55.1, 86.925) -> (56.925, 86.925)